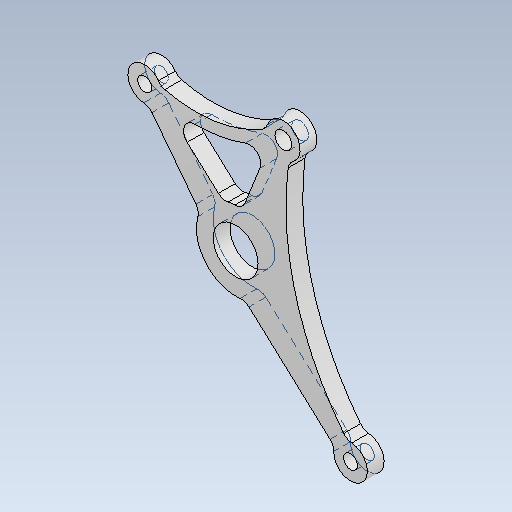
# Autodesk Inventor part: 脚ギアマウントv3
Saved by Autodesk Inventor 2020 (Build 240168000, 168)
## iProperties
Created: 2021-02-23
Part Number: 脚ギアマウントv3
Material: アルミニウム 2014-T4
Document SubType Name: Modeling
Designer: AA19065
Density: 2.8 g/cm^3
Appearance: サテン
Mass: 4.32503 g
Surface Area: 17.5745 cm^2
Volume: 1.54465 cm^3
Author: AA19065
Autodesk Inventor part; units mm, degrees
ref_plane "YZ Plane" through (0, 0, 0) normal (1, 0, 0) x (0, 1, 0)
ref_plane "XZ Plane" through (0, 0, 0) normal (0, 1, 0) x (-1, 0, 0)
ref_plane "XY Plane" through (0, 0, 0) normal (0, 0, 1) x (1, 0, 0)
sketch "スケッチ1" plane through (0, 0, 0) normal (0, 0, 1) x (1, 0, 0)
  circle A0 centre (7.2626, 48.3008) radius 1.25
  circle A1 centre (23.4968, 30.6245) radius 4.005
  circle A2 centre (44, 8.3001) radius 1.25
  line L0 (10.1247, 47.4019) -> (21.2271, 37.2516)
  line L1 (17.0863, 33.4486) -> (7.9152, 45.3726)
  circle A3 centre (23.4968, 30.6245) radius 7.005
  line L2 (41.1378, 9.199) -> (25.1486, 23.817)
  line L3 (30.1394, 28.4007) -> (43.3474, 11.2282)
  circle A4 centre (7.2626, 48.3008) radius 3
  circle A5 centre (44, 8.3001) radius 3
  circle A6 centre (32, 52) radius 1.5
  circle A7 centre (32, 52) radius 3
  line L4 (32, 52) -> (23.4968, 30.6245)
  arc A8 (32, 52) -> (44, 8.3001) centre (80.98, 41.9524) ccw
  arc A9 (7.2626, 48.3008) -> (32, 52) centre (16.4298, 71.5594) ccw
  arc A10 (4.6243, 51.8203) -> (33.4933, 56.1374) centre (16.4298, 71.5594) ccw
  arc A11 (33.2535, 50.5793) -> (44.802, 9.6507) centre (80.98, 41.9524) ccw
  line L5 (33.3938, 51.4456) -> (24.8906, 30.0701)
  line L6 (30.6062, 52.5544) -> (22.103, 31.179)
  point P0 (0, 0)
  point P1 (0, 0)
  point P2 (43.4377, 11.2469)
  point P3 (33.0215, 49.1793)
  point P4 (29.0159, 52.3087)
  point P5 (10.0258, 49.4689)
  point P6 (10.1773, 47.3539)
  point P7 (29.545, 50.2758)
  point P8 (29.6459, 50.1404)
  point P9 (24.6322, 37.5369)
  point P10 (10.1146, 47.3701)
  point P11 (35.2275, 21.7854)
  point P12 (27.4198, 36.428)
  point P13 (31.1236, 45.7388)
  dimension "d0" = 2
  dimension "d1" = 1.5
  dimension "d2" = 1.5
  dimension "d3" = 1.5
  dimension "d4" = 25
  dimension "d5" = 50
  constraints: 14 end point, 12 centre point, 8 point on circle, 2 parallel, 1 coincident, 12 other
  measures "d0" radial gap between concentric circles of A9 A10
  measures "d1" radial gap between concentric circles of A11 A8
  measures "d2" distance between parallel lines of L4 L6
  measures "d3" distance between parallel lines of L4 L5
  measures "d4" radius of A9
  measures "d5" radius of A8
extrude "押し出し1" add sketch "スケッチ1" along normal blind 3 contours A1 L5 A3 L6 | A1 L4 A3 L5 | L6 A3 L4 A1 | L5 A8 L3 A3 | A3 L4 A7 A8 L5 | L6 A7 L4 A3 | L5 A7 A11 A5 L3 A8 | A8 A7 L5 | A3 L1 A4 A9 L0 | L6 A9 A6 L4 A7 | A7 A9 L6 | L4 A6 A8 A7 | L3 A8 A5 L2 A3 | A8 A6 L5 A7 | L3 A5 A8 | L5 A6 L6 A9 A7 A10 | A9 A4 L0 | L0 A4 A10 A7 A9 | L6 A6 A9 | A5 | A4 A10 | A7 A10 | A4 A10
fillet "フィレット1" radius 2 13 edges at (10.1773, 47.3539, 1.5) (10.0258, 49.4689, 1.5) (7.9152, 45.3726, 1.5) (29.0159, 52.3087, 1.5) (29.6459, 50.1404, 1.5) (29.545, 50.2758, 1.5) (33.0215, 49.1793, 1.5) (21.2271, 37.2516, 1.5) (24.6322, 37.5369, 1.5) (17.0863, 33.4486, 1.5) (25.1486, 23.817, 1.5) (43.4377, 11.2469, 1.5) (41.1378, 9.199, 1.5)
